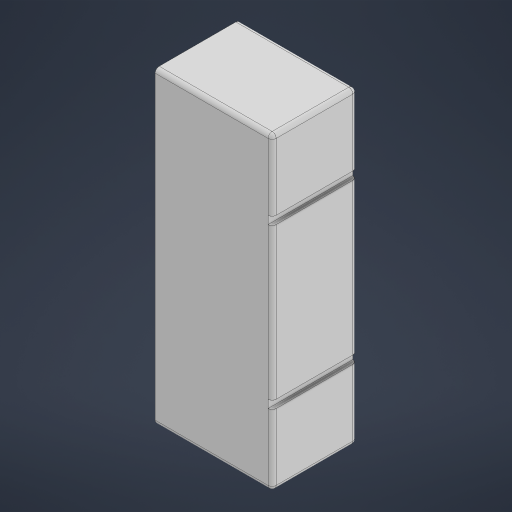
# Autodesk Inventor part: carcasa_lippo
Saved by Autodesk Inventor 2023.1 (Build 271208000, 208)
## iProperties
Created: 2022-12-05
Part Number: carcasa_lippo
Material: Generic
Document SubType Name: Modeling
Designer: amtat
Density: 1 g/cm^3
Appearance: Default
Author: amtat
Autodesk Inventor part; units mm, degrees
ref_plane "YZ Plane" through (0, 0, 0) normal (1, 0, 0) x (0, 1, 0)
ref_plane "XZ Plane" through (0, 0, 0) normal (0, 1, 0) x (-1, 0, 0)
ref_plane "XY Plane" through (0, 0, 0) normal (0, 0, 1) x (1, 0, 0)
sketch "Sketch1" plane through (0, 0, 0) normal (1, 0, 0) x (0, 1, 0)
  line L0 (0, 0) -> (0, -36)
  line L1 (0, 0) -> (36, 0) construction
  line L2 (0, 0) -> (147, 0)
  line L3 (147, 0) -> (147, -36)
  line L4 (147, -36) -> (0, -36)
  line L5 (147, -36) -> (147, -39)
  line L6 (147, -39) -> (-3, -39)
  line L7 (-3, -39) -> (-3, 3)
  line L8 (-3, 3) -> (150, 3)
  line L9 (150, 3) -> (150, -39)
  line L10 (150, -39) -> (147, -39)
  dimension "d0" = 36
  dimension "d1" = 90
  dimension "d2" = 147
  dimension "d3" = 3
  dimension "d4" = 150
  dimension "d5" = 42
  dimension "d6" = 153
  constraints: 22 end point, 7 perpendicular, 3 vertical, 2 point on line, 1 horizontal
  measures "d0" distance of L0.start L0.end
  measures "d1" angle of L0 L1
  measures "d2" distance of L0.start L2.end
  measures "d3" distance of L3.end L5.end
  measures "d4" distance of L5.end L6.end
  measures "d5" distance of L6.end L7.end
  measures "d6" distance of L7.end L8.end
extrude "Extrusion1" add sketch "Sketch1" along normal blind 54
sketch "Sketch2" plane through (54, 0, 0) normal (1, 0, 0) x (0, 0, -1)
  line L0 (39, 150) -> (-3, 150) projected
  line L1 (-3, 150) -> (-3, -3) projected
  line L2 (-3, -3) -> (39, -3) projected
  line L3 (39, -3) -> (39, 150) projected
  line L4 (36, 147) -> (36, 0) projected
  line L5 (36, 0) -> (0, 0) projected
  line L6 (0, 0) -> (0, 147) projected
  line L7 (0, 147) -> (36, 147) projected
extrude "Extrusion2" add sketch "Sketch2" along normal blind 4 contours L3 L2 L1 L0 | L4 L5 L6 L7
sketch "Sketch3" plane through (0, -3, -39) normal (0, -1, 0) x (1, 0, 0)
  line L0 (0, 42) -> (0, 0) projected
  line L1 (0, 0) -> (58, 0) projected
  line L2 (58, 42) -> (58, 0) projected
  line L3 (0, 42) -> (58, 42) projected
  line L4 (0, 0) -> (0, 42) projected
  line L5 (0, 42) -> (0, 39)
  line L6 (0, 3) -> (0, 39) projected
  line L7 (0, 39) -> (10, 39)
  line L8 (0, 39) -> (54, 39) projected
  line L9 (0, 39) -> (10, 39) construction
  line L10 (10, 39) -> (10, 3)
  line L11 (10, 3) -> (0, 3)
  line L12 (0, 3) -> (0, 0)
  dimension "d11" = 10
  dimension "d12" = 0
  dimension "d13" = 36
  constraints: 12 end point, 3 collinear, 1 horizontal, 1 perpendicular
  measures "d11" distance of L5.end L7.end
  measures "d12" distance between parallel lines of L7 L9
  measures "d13" distance of L7.end L10.end
extrude "Extrusion3" cut sketch "Sketch3" against normal blind 4 contours L7 L10 L11 L0
sketch "Sketch4" plane through (58, 0, 0) normal (1, 0, 0) x (0, 0, -1)
  line L0 (-3, 150) -> (-3, -3) projected
  line L1 (-3, -3) -> (39, -3) projected
  line L2 (39, -3) -> (39, 150) projected
  line L3 (39, 150) -> (-3, 150) projected
  line L4 (-3, 150) -> (-3, -3) projected
  line L5 (-3, -3) -> (-3, 32)
  line L6 (-3, 150) -> (-3, 115)
  line L7 (-3, 115) -> (-3, 111)
  line L8 (-3, 111) -> (39, 111)
  line L9 (39, -3) -> (39, 150) projected
  line L10 (39, 111) -> (39, 115)
  line L11 (39, 115) -> (-3, 115)
  line L12 (-3, 32) -> (-3, 36)
  line L13 (-3, 36) -> (39, 36)
  line L14 (39, 36) -> (39, 32)
  line L15 (39, 32) -> (-3, 32)
  point P0 (0, 0)
  dimension "d16" = 35
  dimension "d17" = 35
  dimension "d18" = 4
  dimension "d19" = 4
  dimension "d20" = 4
  constraints: 20 end point, 8 point on line, 3 perpendicular
  measures "d16" distance of L0.end L5.end
  measures "d17" distance of L0.start L6.end
  measures "d18" distance of L6.end L7.end
  measures "d19" distance of L8.end L10.end
  measures "d20" distance of L5.end L12.end
extrude "Extrusion4" cut sketch "Sketch4" against normal blind 2 contours L11 L2 L8 L0 | L13 L2 L15 L0
fillet "Fillet1" radius 2 12 edges at (29, 150, 3) (58, 132.5, 3) (58, 73.5, 3) (58, 150, -18) (58, 132.5, -39) (58, 73.5, -39) (58, 14.5, -39) (58, 14.5, 3) (29, -3, 3) (58, -3, -18) (29, -3, -39) (29, 150, -39)
body "Solid1"
